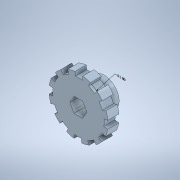
# Autodesk Inventor part: centerPartOfLock
Saved by Autodesk Inventor 2021.2 (Build 252289000, 289)
## iProperties
Created: 2020-11-07
Part Number: centerPartOfLock
Material: PC/ABS Plastic
Document SubType Name: Modeling
Designer: robst
Density: 0.357273 g/cm^3
Appearance: Steel Blue
Author: robst
Autodesk Inventor part; units mm, degrees
ref_plane "YZ Plane" through (0, 0, 0) normal (1, 0, 0) x (0, 1, 0)
ref_plane "XZ Plane" through (0, 0, 0) normal (0, 1, 0) x (-1, 0, 0)
ref_plane "XY Plane" through (0, 0, 0) normal (0, 0, 1) x (1, 0, 0)
sketch "Sketch1" plane through (0, 0, 0) normal (0, 0, 1) x (1, 0, 0)
  circle A0 centre (0, 0) radius 25.4
  dimension "d0" = 50.8
  constraints: 1 centre point, 1 coincident
  measures "d0" diameter of A0
extrude "Extrusion1" add sketch "Sketch1" along normal mid plane 9.525
sketch "Sketch3" plane through (0, 0, 4.7625) normal (0, 0, 1) x (1, 0, 0)
  circle A0 centre (0, 0) radius 25.4 projected
  line L0 (-2.8374, 21.892) -> (-2.8374, 21.8722)
  arc A1 (3.8096, 25.1127) -> (-2.8374, 25.241) centre (0, 0) ccw
  arc A2 (3.3133, 21.8251) -> (-2.466, 21.937) centre (0, 0) ccw
  line L1 (3.3133, 21.8251) -> (3.8096, 25.1127)
  line L2 (-2.466, 21.937) -> (-2.8374, 25.241)
  dimension "d17" = 3.3249
  dimension "d24" = 15
  constraints: 6 end point, 6 point on circle, 2 centre point, 2 coincident, 1 concentric, 1 vertical
  measures "d17" radial gap between concentric circles of A2 A0
  measures "d24" angle of L1 L2
extrude "Extrusion4" cut sketch "Sketch3" against normal blind 9.525 contours L1 A2 L2 A0 picked at (-1.9747, 24.1901)
pattern_circular "Circular Pattern2" count 12 over 360 about axis through (0, 0, -10) along (0, 0, 1) of "Extrusion4"
sketch "Sketch4" plane through (0, 0, -4.7625) normal (0, 0, -1) x (-1, 0, 0)
  circle A0 centre (0, 0) radius 12.7
  dimension "d27" = 25.4
  constraints: 1 centre point, 1 coincident
  measures "d27" diameter of A0
extrude "Extrusion5" add sketch "Sketch4" along normal blind 12.7
sketch "Sketch2" plane through (0, 0, 4.7625) normal (0, 0, 1) x (1, 0, 0)
  line L0 (7.3323, 0) -> (3.6662, -6.35)
  line L1 (3.6662, -6.35) -> (-3.6662, -6.35)
  line L2 (-3.6662, -6.35) -> (-7.3323, 0)
  line L3 (-7.3323, 0) -> (-3.6662, 6.35)
  line L4 (-3.6662, 6.35) -> (3.6662, 6.35)
  line L5 (3.6662, 6.35) -> (7.3323, 0)
  point P0 (0, 0)
  point P1 (0, 0)
  dimension "d23" = 12.7
  constraints: 12 end point, 1 horizontal, 13 other
  measures "d23" distance between parallel lines of L1 L4
extrude "Extrusion2" cut sketch "Sketch2" against normal through all
equation "\"d0\" = externalDiameter"
equation "\"d1\" = thickness"
equation "\"d17\" = heightOfSpline"
equation "\"d18\" = thickness"
equation "\"d23\" = shaftHexSize"
equation "\"externalDiameter\" = 50.8"
equation "\"thickness\" = 9.525"
equation "\"shaftHexSize\" = 12.7"
equation "\"pi\" = 3.141593"
equation "\"heightOfSpline\" = 3.324852"
body "Solid1"
